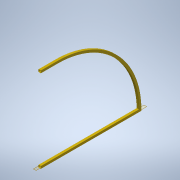
# Autodesk Inventor part: pol luk R1000
Saved by Autodesk Inventor 2021 (Build 250183000, 183)
## iProperties
Created: 2024-04-08
Part Number: pol luk R1000
Material: Steel
Document SubType Name: Modeling
Designer: Michal
Density: 7.85 g/cm^3
Appearance: Glossy - Gold
Author: Michal
Autodesk Inventor part; units mm, degrees
ref_plane "YZ Plane" through (0, 0, 0) normal (1, 0, 0) x (0, 1, 0)
ref_plane "XZ Plane" through (0, 0, 0) normal (0, 1, 0) x (-1, 0, 0)
sketch "Sketch1" plane through (0, 0, 0) normal (0, 1, 0) x (-1, 0, 0)
  line L0 (-12, 14) -> (12, 14) construction
  line L1 (14, 12) -> (14, -12) construction
  line L2 (12, -14) -> (-12, -14) construction
  line L3 (-14, -12) -> (-14, 12) construction
  line L4 (-14, 14) -> (14, -14) construction
  line L5 (14, 14) -> (-14, -14) construction
  arc A0 (14, 12) -> (12, 14) centre (12, 12) ccw construction
  arc A1 (12, -14) -> (14, -12) centre (12, -12) ccw construction
  arc A2 (-14, -12) -> (-12, -14) centre (-12, -12) ccw construction
  arc A3 (-12, 14) -> (-14, 12) centre (-12, 12) ccw construction
  line L6 (-12, -15) -> (12, -15)
  arc A4 (12, -15) -> (15, -12) centre (12, -12) ccw
  line L7 (15, -12) -> (15, 12)
  arc A5 (15, 12) -> (12, 15) centre (12, 12) ccw
  line L8 (12, 15) -> (-12, 15)
  arc A6 (-12, 15) -> (-15, 12) centre (-12, 12) ccw
  line L9 (-15, 12) -> (-15, -12)
  arc A7 (-15, -12) -> (-12, -15) centre (-12, -12) ccw
  line L10 (13, -12) -> (13, 12)
  arc A8 (13, 12) -> (12, 13) centre (12, 12) ccw
  line L11 (12, 13) -> (-12, 13)
  arc A9 (-12, 13) -> (-13, 12) centre (-12, 12) ccw
  line L12 (-13, 12) -> (-13, -12)
  arc A10 (-13, -12) -> (-12, -13) centre (-12, -12) ccw
  line L13 (-12, -13) -> (12, -13)
  arc A11 (12, -13) -> (13, -12) centre (12, -12) ccw
  point P0 (0, 0)
  point P1 (0, 0)
  point P2 (0, 0)
  dimension "d10" = 2
  dimension "depth" = 30
  dimension "width" = 30
  dimension "thickness" = 2
  constraints: 28 end point, 24 point on circle, 12 centre point, 8 point on line, 8 tangent, 6 parallel, 3 equal radius, 3 midpoint, 3 perpendicular, 1 coincident, 1 horizontal, 15 other
  measures "d10" radius of A0
  measures "depth" distance between parallel lines of L6 L8
  measures "width" distance between parallel lines of L9 L7
  measures "thickness" distance between parallel lines of L10 L7
sketch "Sketch3" plane through (0, 0, 0) normal (1, 0, 0) x (0, 1, 0)
  line L0 (0, 0) -> (1200, 0)
  line L1 (0, 0) -> (0, 1000) construction
  line L2 (0, 1000) -> (200, 1000)
  arc A0 (1200, 0) -> (200, 1000) centre (200, 0) ccw
  dimension "d29" = 1200
  dimension "d46" = 1000
  dimension "d47" = 200
  dimension "d48" = 1000
  constraints: 6 end point, 2 horizontal, 2 point on circle, 1 centre point, 1 vertical
  measures "d29" distance of L0.start L0.end
  measures "d46" distance of L0.start L1.end
  measures "d47" distance of L1.end L2.end
  measures "d48" radius of A0
sweep "Sweep1" add profiles "Sketch1" path "Sketch3" path curves L0 A0 L2
sketch "Sketch4" plane through (-15, 0, 12) normal (-1, 0, 0) x (0, 0, 1)
  line L0 (-24, 0) -> (0, 0) projected
  line L1 (-12, 0) -> (-12, 351.1006) construction
  line L2 (988, 0) -> (988, 178.5981) construction
  line L3 (976, 0) -> (1000, 0) projected
  line L4 (1000, 0) -> (976, 0) projected
  point P0 (-12, 50)
  point P1 (-12, 100)
  point P2 (988, 50)
  point P3 (988, 100)
  point P4 (988, 0)
  dimension "d34" = 50
  dimension "d35" = 50
  dimension "d36" = 50
  dimension "d49" = 50
  constraints: 5 point on line, 4 end point, 2 vertical, 1 midpoint
  measures "d34" distance of point (-12, 50) point (-12, 100)
  measures "d35" distance from line of L0 point (-12, 50)
  measures "d36" distance of point (988, 50) point (988, 100)
  measures "d49" distance from line of point (988, 50) L4
hole "Hole2" at (-15, 50, 0) at (-15, 100, 0) at (-15, 50, 1000) at (-15, 100, 1000) direction (1, 0, 0) diameter 9 depth 20.2 tip angle 118
equation "\"d10\" = thickness"
equation "\"d29\" = d46 + d47"
equation "\"d48\" = d46"
body "Solid2"
